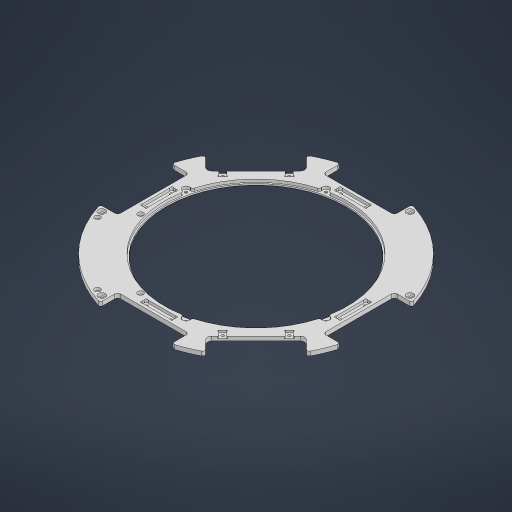
# Autodesk Inventor part: BasePlate
Saved by Autodesk Inventor 2024.2 (Build 282272000, 272)
## iProperties
Created: 2023-12-21
Part Number: BasePlate
Material: 一般
Document SubType Name: Modeling
Designer: Hanaoka
Density: 1 g/cm^3
Appearance: 既定
Author: Hanaoka
Autodesk Inventor part; units mm, degrees
ref_plane "YZ Plane" through (0, 0, 0) normal (1, 0, 0) x (0, 1, 0)
ref_plane "XZ Plane" through (0, 0, 0) normal (0, 1, 0) x (-1, 0, 0)
ref_plane "XY Plane" through (0, 0, 0) normal (0, 0, 1) x (1, 0, 0)
derived "MotorMount_main.ipt"
sketch "モーター固定" plane through (-11, -15, 0) normal (0, -1, 0) x (1, 0, 0)
  circle A0 centre (19.5, 2) radius 0.8
  circle A1 centre (2.5, 2) radius 0.8
  line L0 (22, 0) -> (0, 0)
  line L1 (0, 0) -> (0, 4)
  line L2 (22, 4) -> (0, 4)
  line L3 (22, 0) -> (22, 4)
  circle A2 centre (11, -66) radius 90 construction
  line L4 (2.5, 2) -> (19.5, 2) construction
  line L5 (11, 2) -> (11, -66) construction
  circle A3 centre (11, -66) radius 88
  line L6 (-14, 18.3742) -> (-14, 8)
  line L7 (-12, 6) -> (34, 6)
  line L8 (36, 8) -> (36, 18.3742)
  arc A4 (-14, 8) -> (-12, 6) centre (-12, 8) ccw
  arc A5 (34, 6) -> (36, 8) centre (34, 8) ccw
  line L9 (0, 0) -> (22, 0)
  line L10 (22, 0) -> (22, 4)
  line L11 (22, 4) -> (0, 4)
  line L12 (0, 4) -> (0, 0)
  circle A6 centre (19.5, 2) radius 1
  circle A7 centre (2.5, 2) radius 1
  circle A8 centre (-57, -74.5) radius 1
  line L13 (-59, -77) -> (-55, -77)
  line L14 (-57, -74.5) -> (-57, -57.5) construction
  line L15 (-59, -55) -> (-59, -77)
  line L16 (-55, -55) -> (-59, -55)
  line L17 (-55, -77) -> (-55, -55)
  line L18 (-61, -89) -> (-61, -43)
  circle A9 centre (-57, -57.5) radius 1
  arc A10 (-63, -91) -> (-61, -89) centre (-63, -89) ccw
  line L19 (-63, -41) -> (-73.3742, -41)
  arc A11 (-61, -43) -> (-63, -41) centre (-63, -43) ccw
  line L20 (-73.3742, -91) -> (-63, -91)
  circle A12 centre (19.5, -134) radius 1
  line L21 (22, -136) -> (22, -132)
  line L22 (19.5, -134) -> (2.5, -134) construction
  line L23 (0, -136) -> (22, -136)
  line L24 (0, -132) -> (0, -136)
  line L25 (22, -132) -> (0, -132)
  line L26 (34, -138) -> (-12, -138)
  circle A13 centre (2.5, -134) radius 1
  arc A14 (36, -140) -> (34, -138) centre (34, -140) ccw
  line L27 (-14, -140) -> (-14, -150.3742)
  arc A15 (-12, -138) -> (-14, -140) centre (-12, -140) ccw
  line L28 (36, -150.3742) -> (36, -140)
  circle A16 centre (79, -57.5) radius 1
  line L29 (81, -55) -> (77, -55)
  line L30 (79, -57.5) -> (79, -74.5) construction
  line L31 (81, -77) -> (81, -55)
  line L32 (77, -77) -> (81, -77)
  line L33 (77, -55) -> (77, -77)
  line L34 (83, -43) -> (83, -89)
  circle A17 centre (79, -74.5) radius 1
  arc A18 (85, -41) -> (83, -43) centre (85, -43) ccw
  line L35 (85, -91) -> (95.3742, -91)
  arc A19 (83, -89) -> (85, -91) centre (85, -89) ccw
  line L36 (95.3742, -41) -> (85, -41)
  arc A20 (78.4142, -55) -> (77, -56.4142) centre (77.7071, -55.7071) ccw
  line L37 (77.7071, -55.7071) -> (77.7071, -55) construction
  line L38 (77.7071, -55.7071) -> (77, -55.7071) construction
  line L39 (77.7071, -55.7071) -> (77, -55) construction
  line L40 (80.2929, -55) -> (80.2929, -55.7071) construction
  line L41 (80.2929, -55.7071) -> (81, -55.7071) construction
  line L42 (77.7071, -77) -> (77.7071, -76.2929) construction
  line L43 (77.7071, -76.2929) -> (77, -76.2929) construction
  line L44 (81, -76.2929) -> (80.2929, -76.2929) construction
  line L45 (80.2929, -76.2929) -> (80.2929, -77) construction
  line L46 (81, -77) -> (80.2929, -76.2929) construction
  line L47 (77.7071, -76.2929) -> (77, -77) construction
  line L48 (81, -55) -> (80.2929, -55.7071) construction
  arc A21 (81, -56.4142) -> (79.5858, -55) centre (80.2929, -55.7071) ccw
  arc A22 (79.5858, -77) -> (81, -75.5858) centre (80.2929, -76.2929) ccw
  arc A23 (77, -75.5858) -> (78.4142, -77) centre (77.7071, -76.2929) ccw
  arc A24 (20.5858, 0) -> (22, 1.4142) centre (21.2929, 0.7071) ccw
  arc A25 (22, 2.5858) -> (20.5858, 4) centre (21.2929, 3.2929) ccw
  arc A26 (0, 1.4142) -> (1.4142, 0) centre (0.7071, 0.7071) ccw
  arc A27 (1.4142, 4) -> (0, 2.5858) centre (0.7071, 3.2929) ccw
  arc A28 (-55, -56.4142) -> (-56.4142, -55) centre (-55.7071, -55.7071) ccw
  arc A29 (-57.5858, -55) -> (-59, -56.4142) centre (-58.2929, -55.7071) ccw
  arc A30 (-56.4142, -77) -> (-55, -75.5858) centre (-55.7071, -76.2929) ccw
  arc A31 (-59, -75.5858) -> (-57.5858, -77) centre (-58.2929, -76.2929) ccw
  arc A32 (1.4142, -132) -> (0, -133.4142) centre (0.7071, -132.7071) ccw
  arc A33 (0, -134.5858) -> (1.4142, -136) centre (0.7071, -135.2929) ccw
  arc A34 (22, -133.4142) -> (20.5858, -132) centre (21.2929, -132.7071) ccw
  arc A35 (20.5858, -136) -> (22, -134.5858) centre (21.2929, -135.2929) ccw
  point P0 (11, 0)
  point P1 (-14, 6)
  point P2 (36, 6)
  point P3 (-57, -66)
  point P4 (-61, -91)
  point P5 (-61, -41)
  point P6 (11, -134)
  point P7 (36, -138)
  point P8 (-14, -138)
  point P9 (79, -66)
  point P10 (83, -41)
  point P11 (83, -91)
  point P12 (22, -134.5858)
  point P13 (20.5858, -136)
  point P14 (1.4142, -136)
  point P15 (0, -134.5858)
  point P16 (0, -133.4142)
  point P17 (1.4142, -132)
  point P18 (20.5858, -132)
  point P19 (-59, -75.5858)
  point P20 (-59, -56.4142)
  point P21 (-57.5858, -55)
  point P22 (-55, -75.5858)
  point P23 (0, 2.5858)
  point P24 (1.4142, 4)
  point P25 (20.5858, 4)
  point P26 (22, 2.5858)
  point P27 (22, 1.4142)
  point P28 (20.5858, 0)
  point P29 (1.4142, 0)
  point P30 (0, 1.4142)
  dimension "d4" = 180
  dimension "d5" = 68
  dimension "d6" = 176
  dimension "d11" = 2
  dimension "d12" = 50
  dimension "d13" = 2
  dimension "d14" = 2
  dimension "d17" = 360
  dimension "d31" = 1
  dimension "d32" = 1
  dimension "d35" = 360
  measures "d4" diameter of A2
  measures "d5" distance of L5.start L5.end
  measures "d6" diameter of A3
  measures "d11" distance between parallel lines of L7 L2
  measures "d12" distance of point (-14, 6) point (36, 6)
  measures "d13" radius of A4
  measures "d14" diameter of A7
  measures "d31" radius of A20
  measures "d32" distance of L37.start L29.end
extrude "押し出し2" add sketch "モーター固定" along normal blind 1 contours A24 L0 | L0 L1 L2 L3 | L3 A24 | A26 L0 | L3 A25 | A26 L1 | L2 A25 | A27 L1 | L2 A27 | L36 A18 L34 A19 L35 A3 L28 A14 L26 A15 L27 L20 A10 L18 A11 L19 L6 A4 L7 A5 L8 | A6 | A7 | L15 L16 L17 L13 | A31 L15 | L13 A31 | L13 A30 | A29 L15 | L17 A30 | A29 L16 | L17 A28 | A28 L16 | L23 L24 L25 L21 | A35 L23 | L21 A35 | L21 A34 | A33 L23 | L25 A34 | A33 L24 | L25 A32 | A32 L24 | L31 L32 L33 L29 | A21 L31 | L29 A21 | L29 A20 | A22 L31 | L33 A20 | A22 L32 | L33 A23 | A23 L32
extrude "押し出し3" add sketch "モーター固定" against normal blind 2 contours L36 A18 L34 A19 L35 A3 L28 A14 L26 A15 L27 L20 A10 L18 A11 L19 L6 A4 L7 A5 L8
fillet "フィレット1" radius 1.5 8 edges at (-84.3742, -14.5, -41) (-25, -14.5, 18.3742) (25, -14.5, 18.3742) (84.3742, -14.5, -41) (84.3742, -14.5, -91) (25, -14.5, -150.3742) (-25, -14.5, -150.3742) (-84.3742, -14.5, -91)
sketch "溝切り" plane through (-23, -13, 6) normal (0, 1, 0) x (1, 0, 0)
  circle A0 centre (102.5487, 100.5) radius 2.5
  line L0 (97, 97) -> (105.3408, 97) projected
  arc A1 (106.7686, 98.9595) -> (49.9595, 155.7686) centre (23, 72) ccw projected
  circle A2 centre (102.5487, 100.5) radius 3.5 construction
  line L1 (85.2254, 134.2254) -> (-39.2254, 9.7746) construction
  arc A3 (-60.7686, 45.0405) -> (-3.9595, -11.7686) centre (23, 72) ccw projected
  circle A4 centre (51.5, 151.5487) radius 2.5
  circle A5 centre (51.5, 151.5487) radius 3.5 construction
  line L2 (-39.2254, 134.2254) -> (85.2254, 9.7746) construction
  arc A6 (49.9595, -11.7686) -> (106.7686, 45.0405) centre (23, 72) ccw projected
  arc A7 (-3.9595, 155.7686) -> (-60.7686, 98.9595) centre (23, 72) ccw projected
  circle A8 centre (-5.5, -7.5487) radius 2.5
  circle A9 centre (-5.5, -7.5487) radius 3.5 construction
  circle A10 centre (-56.5487, 43.5) radius 3.5 construction
  circle A11 centre (-56.5487, 43.5) radius 2.5
  circle A12 centre (102.5487, 100.5) radius 1.3
  circle A13 centre (51.5, 151.5487) radius 1.3
  circle A14 centre (-56.5487, 43.5) radius 1.3
  circle A15 centre (-5.5, -7.5487) radius 1.3
  circle A16 centre (23, 72) radius 63
  line L3 (-54.3392, 113.9839) -> (-46.9146, 106.5593)
  line L4 (-42.672, 106.5593) -> (-11.5593, 137.672)
  line L5 (-11.5593, 141.9146) -> (-18.9839, 149.3392)
  arc A17 (-46.9146, 106.5593) -> (-42.672, 106.5593) centre (-44.7933, 108.6806) ccw
  arc A18 (-11.5593, 137.672) -> (-11.5593, 141.9146) centre (-13.6806, 139.7933) ccw
  circle A19 centre (-41.9648, 136.9648) radius 21 construction
  line L6 (64.9839, -5.3392) -> (57.5593, 2.0854)
  line L7 (57.5593, 6.328) -> (88.672, 37.4407)
  line L8 (92.9146, 37.4407) -> (100.3392, 30.0161)
  arc A20 (57.5593, 6.328) -> (57.5593, 2.0854) centre (59.6806, 4.2067) ccw
  arc A21 (92.9146, 37.4407) -> (88.672, 37.4407) centre (90.7933, 35.3194) ccw
  circle A22 centre (8.2657, 135.8212) radius 2.5 construction
  circle A23 centre (8.2657, 135.8212) radius 1
  line L9 (8.2657, 135.8212) -> (23, 72) construction
  arc A24 (10.7016, 136.3836) -> (5.8298, 135.2589) centre (8.2657, 135.8212) ccw
  line L10 (5.8298, 135.2589) -> (6.4033, 132.7746)
  line L11 (10.7016, 136.3836) -> (11.2752, 133.8993)
  circle A25 centre (-40.8212, 86.7343) radius 2.5 construction
  circle A26 centre (-40.8212, 86.7343) radius 1
  arc A27 (-40.2589, 89.1702) -> (-41.3836, 84.2984) centre (-40.8212, 86.7343) ccw
  line L12 (-40.2589, 89.1702) -> (-37.7746, 88.5967)
  line L13 (-41.3836, 84.2984) -> (-38.8993, 83.7248)
  circle A28 centre (86.8212, 57.2657) radius 2.5 construction
  circle A29 centre (86.8212, 57.2657) radius 1
  arc A30 (86.2589, 54.8298) -> (87.3836, 59.7016) centre (86.8212, 57.2657) ccw
  line L14 (86.2589, 54.8298) -> (83.7746, 55.4033)
  line L15 (87.3836, 59.7016) -> (84.8993, 60.2752)
  line L16 (35.2984, 7.6164) -> (34.7248, 10.1007)
  line L17 (40.1702, 8.7411) -> (39.5967, 11.2254)
  circle A31 centre (37.7343, 8.1788) radius 2.5 construction
  circle A32 centre (37.7343, 8.1788) radius 1
  arc A33 (35.2984, 7.6164) -> (40.1702, 8.7411) centre (37.7343, 8.1788) ccw
  circle A34 centre (23, 72) radius 64
  point P0 (23, 6)
  point P1 (-44.7933, 104.4379)
  point P2 (-9.4379, 139.7933)
  point P3 (83.7746, 55.4033)
  point P4 (-37.7746, 88.5967)
  point P5 (-39.8745, 83.95)
  point P6 (34.95, 9.1255)
  point P7 (39.8218, 10.2503)
  point P8 (84.7497, 55.1782)
  point P9 (85.8745, 60.05)
  point P10 (11.05, 134.8745)
  point P11 (6.1782, 133.7497)
  point P12 (-38.7497, 88.8218)
  dimension "d20" = 5
  dimension "d22" = 7
  dimension "d23" = 2.6
  dimension "d28" = 126
  dimension "d37" = 50
  dimension "d38" = 3
  dimension "d39" = 42
  dimension "d40" = 13.5
  dimension "d45" = 2
  dimension "d46" = 5
  dimension "d47" = 32
  dimension "d48" = 1
  constraints: 35 symmetric about line, 34 end point, 31 centre point, 24 point on circle, 18 coincident, 11 tangent, 6 parallel, 5 equal radius, 5 point on line, 1 midpoint, 17 other
  measures "d20" diameter of A0
  measures "d22" diameter of A2
  measures "d23" diameter of A12
  measures "d28" diameter of A16
  measures "d37" distance of point (-44.793, 104.438) point (-9.438, 139.793)
  measures "d38" radius of A17
  measures "d39" diameter of A19
  measures "d40" distance from line of L5.end L4
  measures "d45" diameter of A23
  measures "d46" diameter of A22
  measures "d47" angle of L2 L9
  measures "d48" radial gap between concentric circles of A16 A34
extrude "押し出し4" cut sketch "溝切り" against normal up to surface (3 mm away) contours A12 | A13 | A14 | A15
extrude "押し出し5" cut sketch "溝切り" against normal blind 2 contours A0 | A4 | A8 | A11 | A15 | A16 | A16 L11 A34 L15 | A16 L10 A34 L11 | L15 A34 L14 A16 | A16 L12 A34 L10 | A34 L10 A24 L11 | L14 A34 L17 A16 | L15 A30 L14 A34 | A16 L13 A34 L12 | L17 A34 L16 A16 | A16 L16 A34 L13 | A34 L13 A27 L12 | L17 A33 L16 A34
extrude "押し出し6" cut sketch "溝切り" against normal up to surface (3 mm away) contours L6 A20 L7 A21 L8 A6 | L5 A18 L4 A17 L3 A7 | A16 | A23 | A26 | A29 | A32
fillet "フィレット2" radius 1.5 4 edges at (-77.3392, -14.5, -107.9839) (-41.9839, -14.5, -143.3392) (41.9839, -14.5, 11.3392) (77.3392, -14.5, -24.0161)
fillet "フィレット3" radius 1.5 8 edges at (-61.7497, -14, -82.8218) (-62.8745, -14, -77.95) (-16.8218, -14, -127.7497) (-11.95, -14, -128.8745) (62.8745, -14, -54.05) (61.7497, -14, -49.1782) (11.95, -14, -3.1255) (16.8218, -14, -4.2503)
sketch "シャフト用はめ穴" plane through (-23, -13, -138) normal (0, 1, 0) x (1, 0, 0)
  circle A0 centre (-54.5262, -105.6146) radius 1
  circle A1 centre (-54.5262, -105.6146) radius 2
  circle A2 centre (-41.4205, -88.5) radius 2
  circle A3 centre (-41.4205, -88.5) radius 1
  circle A4 centre (-56.5487, -100.5) radius 2.5 projected
  circle A5 centre (23, -72) radius 63 projected
  arc A6 (-56.5487, -100.5) -> (-54.5262, -105.6146) centre (23, -72) ccw construction
  line L0 (85.2254, -9.7746) -> (-39.2254, -134.2254) construction
  line L1 (-39.2254, -9.7746) -> (85.2254, -134.2254) construction
  circle A7 centre (-10.6146, -149.5262) radius 1
  circle A8 centre (-10.6146, -149.5262) radius 2
  circle A9 centre (-41.4205, -88.5) radius 2.5 construction
  arc A10 (-40.1225, -61.4382) -> (33.5618, -135.1225) centre (23, -72) ccw projected
  line L2 (-44.4142, -83) -> (-45.5858, -83) projected
  circle A11 centre (6.5, -136.4205) radius 2
  circle A12 centre (6.5, -136.4205) radius 1
  circle A13 centre (6.5, -136.4205) radius 2.5 construction
  circle A14 centre (56.6146, 5.5262) radius 1
  circle A15 centre (56.6146, 5.5262) radius 2
  circle A16 centre (39.5, -7.5795) radius 2
  circle A17 centre (39.5, -7.5795) radius 1
  circle A18 centre (100.5262, -38.3854) radius 1
  circle A19 centre (100.5262, -38.3854) radius 2
  circle A20 centre (87.4205, -55.5) radius 2
  circle A21 centre (87.4205, -55.5) radius 1
  point P0 (23, -138)
  dimension "d50" = 2
  dimension "d51" = 4
  dimension "d52" = 1
  dimension "d53" = 5
  dimension "d54" = 3
  constraints: 19 centre point, 13 symmetric about line, 12 coincident, 2 equal radius, 2 point on circle, 1 tangent, 13 other
  measures "d50" diameter of A0
  measures "d51" diameter of A1
  measures "d53" diameter of A9
  measures "d54" distance edge to line of A9 L2
extrude "押し出し7" cut sketch "シャフト用はめ穴" against normal up to surface (2 mm away) contours A0 | A1 | A2 | A3 | A7 | A8 | A11 | A12
extrude "押し出し8" cut sketch "シャフト用はめ穴" against normal up to surface (3 mm away) contours A0 | A3 | A7 | A12
sketch "キッカー用はめあい" plane through (-23, -13, -138) normal (0, 1, 0) x (1, 0, 0)
  circle A0 centre (83.0151, -108.6806) radius 1
  circle A1 centre (59.6806, -132.0151) radius 1
  line L0 (88.672, -106.5593) -> (57.5593, -137.672) projected
  line L1 (73.1156, -122.1156) -> (68.2548, -117.2548) construction
  line L2 (57.5593, -137.672) -> (88.672, -106.5593) projected
  arc A2 (41.1782, -133.3641) -> (84.3641, -90.1782) centre (23, -72) ccw projected
  line L3 (59.6806, -132.0151) -> (83.0151, -108.6806) construction
  line L4 (86.1971, -109.0341) -> (82.6615, -105.4986)
  line L5 (82.6615, -105.4986) -> (79.8331, -108.327)
  line L6 (79.8331, -108.327) -> (83.3687, -111.8626)
  circle A3 centre (83.0151, -108.6806) radius 2 construction
  line L7 (60.0341, -135.1971) -> (56.4986, -131.6615)
  line L8 (56.4986, -131.6615) -> (59.327, -128.8331)
  line L9 (59.327, -128.8331) -> (62.8626, -132.3687)
  arc A4 (83.3687, -106.2057) -> (82.6615, -105.4986) centre (83.0151, -105.8521) ccw
  line L10 (82.6615, -105.4986) -> (83.0151, -105.8521)
  line L11 (79.8331, -108.327) -> (80.1867, -108.6806)
  arc A5 (79.8331, -108.327) -> (80.5402, -109.0341) centre (80.1867, -108.6806) ccw
  arc A6 (56.4986, -131.6615) -> (57.2057, -132.3687) centre (56.8521, -132.0151) ccw
  arc A7 (60.0341, -129.5402) -> (59.327, -128.8331) centre (59.6806, -129.1867) ccw
  line L12 (-21.5477, -116.5477) -> (67.5477, -27.4523) construction
  circle A8 centre (23, -72) radius 63 projected
  circle A9 centre (-13.6806, -11.9849) radius 1
  circle A10 centre (-37.0151, -35.3194) radius 1
  line L13 (-27.1156, -21.8844) -> (-22.2548, -26.7452) construction
  line L14 (-37.0151, -35.3194) -> (-13.6806, -11.9849) construction
  line L15 (-14.0341, -8.8029) -> (-10.4986, -12.3385)
  line L16 (-10.4986, -12.3385) -> (-13.327, -15.1669)
  line L17 (-13.327, -15.1669) -> (-16.8626, -11.6313)
  circle A11 centre (-13.6806, -11.9849) radius 2 construction
  line L18 (-40.1971, -34.9659) -> (-36.6615, -38.5014)
  line L19 (-36.6615, -38.5014) -> (-33.8331, -35.673)
  line L20 (-33.8331, -35.673) -> (-37.3687, -32.1374)
  arc A12 (-10.4986, -12.3385) -> (-11.2057, -11.6313) centre (-10.8521, -11.9849) ccw
  line L21 (-10.4986, -12.3385) -> (-10.8521, -11.9849)
  line L22 (-13.327, -15.1669) -> (-13.6806, -14.8133)
  arc A13 (-14.0341, -14.4598) -> (-13.327, -15.1669) centre (-13.6806, -14.8133) ccw
  arc A14 (-37.3687, -37.7943) -> (-36.6615, -38.5014) centre (-37.0151, -38.1479) ccw
  arc A15 (-33.8331, -35.673) -> (-34.5402, -34.9659) centre (-34.1867, -35.3194) ccw
  line L23 (-40.1971, -34.9659) -> (-37.3687, -32.1374)
  line L24 (-42.672, -37.4407) -> (-11.5593, -6.328) projected
  line L25 (-16.8626, -11.6313) -> (-14.0341, -8.8029)
  point P0 (23, -138)
  point P1 (56.4986, -131.6615)
  point P2 (57.2057, -132.3687)
  point P3 (-13.327, -15.1669)
  point P4 (-36.6615, -38.5014)
  point P5 (-33.8331, -35.673)
  point P6 (-34.5402, -34.9659)
  point P7 (-37.3687, -37.7943)
  dimension "d59" = 2
  dimension "d60" = 33
  dimension "d61" = 2.5
  dimension "d62" = 4
  dimension "d63" = 5
  dimension "d68" = 0.5
  dimension "d69" = 0.5
  constraints: 46 end point, 37 symmetric about line, 19 point on circle, 14 centre point, 14 point on line, 6 coincident, 4 parallel, 3 perpendicular, 2 collinear, 2 equal radius, 2 midpoint, 2 tangent, 10 other
  measures "d59" diameter of A0
  measures "d60" distance of L3.start L3.end
  measures "d61" distance between parallel lines of L0 L3
  measures "d62" diameter of A3
  measures "d63" distance of L4.start L4.end
  measures "d68" distance of L4.end L10.end
  measures "d69" radius of A4
extrude "押し出し9" cut sketch "キッカー用はめあい" against normal blind 1.5 contours A0 | A1 | L0 L6 L5 L4 | L4 A4 | A5 L6 | L0 L7 L8 L9 | L9 A7 | A6 L7 | A9 | A10 | L15 L16 L17 L24 | A12 L15 | L17 A13 | L23 L20 L19 L18 | L18 A14 | A15 L20
extrude "押し出し10" cut sketch "キッカー用はめあい" against normal up to surface (3 mm away) contours A0 | A1 | A9 | A10
fillet "フィレット4" radius 0.5 8 edges at (37.0341, -13.75, -2.8029) (39.8626, -13.75, -5.6313) (60.3687, -13.75, -26.1374) (63.1971, -13.75, -28.9659) (-63.1971, -13.75, -103.0341) (-60.3687, -13.75, -105.8626) (-39.8626, -13.75, -126.3687) (-37.0341, -13.75, -129.1971)
